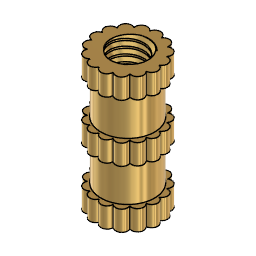
M3_10_mm_threaded_brass_insert (Autodesk Fusion 360 design; units mm, degrees)
part number: 2026-06-20-09-24-02-047
Autodesk Fusion 360 part; units mm, degrees
sketch "Brass thread outline" plane through (0, 0, 0) normal (0, 0, 1) x (1, 0, 0)
  circle A0 centre (0, 0) radius 2
  dimension "d4" = 4
  constraint coincident A0.centre origin
  measures "d4" diameter of A0
extrude "Extrude1" add sketch "Brass thread outline" along normal blind 10
sketch "Ridges" plane through (0, 0, 10) normal (0, 0, 1) x (-1, 0, 0)
  circle A0 centre (0, 0) radius 2
  circle A1 centre (0, 0) radius 2.45
  circle A2 centre (-0.0001, -2) radius 0.45
  circle A3 centre (0.8134, -1.8271) radius 0.45
  circle A4 centre (1.4862, -1.3383) radius 0.45
  circle A5 centre (1.9021, -0.6181) radius 0.45
  circle A6 centre (1.9891, 0.209) radius 0.45
  circle A7 centre (1.7321, 0.9999) radius 0.45
  circle A8 centre (1.1757, 1.618) radius 0.45
  circle A9 centre (0.4159, 1.9563) radius 0.45
  circle A10 centre (-0.4157, 1.9563) radius 0.45
  circle A11 centre (-1.1755, 1.6181) radius 0.45
  circle A12 centre (-1.732, 1.0001) radius 0.45
  circle A13 centre (-1.989, 0.2092) radius 0.45
  circle A14 centre (-1.9021, -0.6179) radius 0.45
  circle A15 centre (-1.4864, -1.3382) radius 0.45
  circle A16 centre (-0.8136, -1.8271) radius 0.45
  dimension "d8" = 4.9
  dimension "d29" = 0.0001
  dimension "d31" = 360
  constraint coincident A0.centre A1.centre
  constraint coincident A0 A2.centre
  constraint tangent A1 A2
  measures "d8" diameter of A1
  measures "d29" horizontal distance of A0.centre A2.centre
extrude "Extrude2" add sketch "Ridges" against normal blind 1.5 contours A0 A5 A6 A7 | A0 A5 A6 A7 | A0 A6 A7 | A0 A6 A7 | A0 A5 A6 | A0 A5 A6 | A0 A6 A7 A8 | A0 A6 A7 A8 | A2 A3 A4 A5 A6 A7 A8 A9 A10 A11 A12 A13 A14 A15 A16 | A0 A4 A5 A6 | A0 A4 A5 A6 | A0 A7 A8 | A0 A7 A8 | A0 A7 A8 A9 | A0 A4 A5 | A0 A4 A5 | A0 A3 A4 A5 | A0 A7 A8 A9 | A0 A8 A9 A10 | A0 A8 A9 | A0 A3 A4 A5 | A0 A2 A3 A4 | A0 A3 A4 | A0 A8 A9 | A0 A8 A9 A10 | A0 A9 A10 A11 | A0 A9 A10 | A0 A3 A4 | A0 A2 A3 A16 | A0 A2 A3 | A0 A2 A3 A4 | A0 A9 A10 | A0 A9 A10 A11 | A0 A10 A11 A12 | A0 A10 A11 | A0 A2 A3 | A0 A2 A16 | A0 A2 A15 A16 | A0 A2 A3 A16 | A0 A10 A11 | A0 A10 A11 A12 | A0 A2 A15 A16 | A0 A2 A16 | A0 A14 A15 A16 | A0 A15 A16 | A0 A11 A12 | A0 A11 A12 | A0 A11 A12 A13 | A0 A15 A16 | A0 A14 A15 A16 | A0 A11 A12 A13 | A0 A13 A14 A15 | A0 A14 A15 | A0 A14 A15 | A0 A12 A13 | A0 A12 A13 | A0 A12 A13 A14 | A0 A12 A13 A14 | A0 A13 A14 A15 | A0 A13 A14 | A0 A13 A14
pattern_linear "R-Pattern1" count 3 spacing 4.25 along (0, 0, -1) of "Extrude2"
sketch "Thread hole" plane through (0, 0, 10) normal (0, 0, 1) x (-1, 0, 0)
  circle A0 centre (0, 0) radius 1.5
  arc A1 (0.4424, -2.0818) -> (1.2509, -1.7219) centre (0.8134, -1.8271) ccw
  arc A2 (1.2509, -1.7219) -> (1.8431, -1.0642) centre (1.4862, -1.3383) ccw
  arc A3 (1.8431, -1.0642) -> (2.1166, -0.2226) centre (1.9021, -0.6181) ccw
  arc A4 (2.1166, -0.2226) -> (2.0242, 0.6576) centre (1.9891, 0.209) ccw
  arc A5 (2.0242, 0.6576) -> (1.5817, 1.424) centre (1.7321, 0.9999) ccw
  arc A6 (1.5817, 1.424) -> (0.8658, 1.9443) centre (1.1757, 1.618) ccw
  arc A7 (0.8658, 1.9443) -> (0.0001, 2.1283) centre (0.4159, 1.9563) ccw
  arc A8 (0.0001, 2.1283) -> (-0.8656, 1.9444) centre (-0.4157, 1.9563) ccw
  arc A9 (-0.8656, 1.9444) -> (-1.5816, 1.4242) centre (-1.1755, 1.6181) ccw
  arc A10 (-1.5816, 1.4242) -> (-2.0241, 0.6578) centre (-1.732, 1.0001) ccw
  arc A11 (-2.0241, 0.6578) -> (-2.1167, -0.2224) centre (-1.989, 0.2092) ccw
  arc A12 (-2.1167, -0.2224) -> (-1.8432, -1.0641) centre (-1.9021, -0.6179) ccw
  arc A13 (-1.8432, -1.0641) -> (-1.2511, -1.7218) centre (-1.4864, -1.3382) ccw
  arc A14 (-1.2511, -1.7218) -> (-0.4426, -2.0818) centre (-0.8136, -1.8271) ccw
  arc A15 (-0.4426, -2.0818) -> (0.4424, -2.0818) centre (-0.0001, -2) ccw
  dimension "d11" = 3
  constraint coincident A0.centre origin
  measures "d11" diameter of A0
extrude "Extrude3" cut sketch "Thread hole" against normal blind 10 contours A0
thread "Thread2" "ISO Metric profile 3.0 M3x0.5 M3x0.5 6H" major diameter 3.086 minor diameter 2.529 pitch 0.5 angle 60 modelled right hand crest width 0.1368 on face at (-1.4981, 0.0748, 3.3333) crest through (-1.2645, 0, 9.875)
equation "outer_diameter = 4 mm" comment "The outer diameter of the non-ridged parts."
equation "hole_diameter = 3 mm" comment "The thread diameter of the brass insert. 3 mm for this M3 insert."
equation "height = 10 mm" comment "The height of the brass thread insert. 10 mm for this model."
equation "d4 = outer_diameter"
equation "d5 = height"
equation "ridge_diameter = 4.9 mm" comment "The outer diameter of the ridged parts."
equation "d8 = ridge_diameter"
equation "d9 = -ridge_height"
equation "d11 = hole_diameter"
equation "d12 = -height"
equation "number_of_ridges = 3" comment "The number of ridges to have along the outside."
equation "d23 = number_of_ridges"
equation "d25 = -ridge_pattern_length"
equation "ridge_pattern_length = height - ridge_height" comment "The distance to use for the rectangular pattern that repeats the ridges."
equation "ridge_height = 1.5 mm" comment "The height of the individual ridges."
named bodies: "M3 10 mm Threaded Brass Insert"
